Autodesk Fusion 360 part; units mm, degrees
note: some values were not read from the file. Set by a fixed rule: which sketch regions a step uses.
(part 4 of 4)
sketch "Sketch1 (7)" plane through (0, 0, 0) normal (0, 0, 1) x (1, 0, 0) in component "Top/Bottom (1)"
  line L0 (0, 0) -> (160, 0)
  line L1 (160, 0) -> (160, 54)
  line L2 (160, 54) -> (0, 54)
  line L3 (0, 54) -> (0, 0)
  line L4 (0, 51) -> (160, 51) construction
  line L5 (160, 51) -> (160, 48) construction
  line L6 (160, 48) -> (0, 48) construction
  line L7 (0, 48) -> (0, 51) construction
  line L8 (0, 3) -> (160, 3) construction
  line L9 (160, 3) -> (160, 6) construction
  line L10 (160, 6) -> (0, 6) construction
  line L11 (0, 6) -> (0, 3) construction
  line L12 (10, 48) -> (150, 48) construction
  line L13 (150, 48) -> (150, 38) construction
  line L14 (150, 38) -> (10, 38) construction
  line L15 (10, 38) -> (10, 48) construction
  line L16 (0, 38) -> (160, 38) construction
  line L17 (160, 38) -> (160, 36) construction
  line L18 (160, 36) -> (0, 36) construction
  line L19 (0, 36) -> (0, 38) construction
  line L20 (80, 54) -> (80, 0) construction
  point P0 (80, 51)
  point P1 (80, 48)
  point P2 (80, 38)
  point P3 (80, 38)
  point P4 (80, 6)
  dimension "d101_1" = 160
  dimension "d102_1" = 3
  dimension "d103_1" = 3
  dimension "d104_1" = 10
  dimension "d105_1" = 2
  dimension "d106_1" = 140
  dimension "d107_1" = 30
  dimension "d108_1" = 3
  dimension "d109_1" = 3
  constraint horizontal L0
  constraint vertical L1
  constraint horizontal L2
  constraint vertical L3
  constraint coincident L0.start L3.end
  constraint horizontal L4
  constraint vertical L5
  constraint horizontal L6
  constraint vertical L7
  constraint horizontal L8
  constraint vertical L9
  constraint horizontal L10
  constraint vertical L11
  constraint horizontal L12
  constraint vertical L13
  constraint horizontal L14
  constraint vertical L15
  constraint horizontal L16
  constraint vertical L17
  constraint horizontal L18
  constraint vertical L19
  constraint midpoint L2 L20.start
  constraint midpoint L0 L20.end
  constraint midpoint L4 P0
  constraint midpoint L12 P1
  constraint midpoint L16 P3
  constraint midpoint L14 P3
  constraint coincident L20 P0
  constraint coincident P3 P2
  constraint midpoint L10 P4
  constraint coincident L20 P4
  constraint coincident L3 L4.start
  constraint coincident L20 P3
  constraint coincident L6 P1
  constraint coincident L3 L18.end
  constraint coincident L3 L8.start
  measures "d101_1" distance of L17 L19
  measures "d102_1" distance of L2 L4
  measures "d103_1" distance of L4 L6
  measures "d104_1" distance of L12.start L14.end
  measures "d105_1" distance of L16.start L18.end
  measures "d106_1" distance of L13 L15
  measures "d107_1" distance of L10 L18
  measures "d108_1" distance of L8 L10
  measures "d109_1" distance of L0 L8
extrude "Extrude1''''''" add sketch "Sketch1 (7)" along normal blind 10 separate body makes body 7 in component "Top/Bottom (1)"
sketch "Sketch2 (5)" plane through (0, 0, 10) normal (0, 0, 1) x (-1, 0, 0) in component "Top/Bottom (1)"
  line L0 (0, -54) -> (0, 0)
  line L1 (0, 0) -> (-160, 0)
  line L2 (-160, 0) -> (-160, -54)
  line L3 (-160, -54) -> (0, -54)
  line L4 (0, -3) -> (-160, -3)
  line L5 (-160, -6) -> (0, -6)
  line L6 (-160, -48) -> (0, -48)
  line L7 (0, -51) -> (-160, -51)
  line L8 (-79, -48) -> (-81, -48)
  line L9 (-81, -48) -> (-81, -38)
  line L10 (-81, -38) -> (-79, -38)
  line L11 (-79, -38) -> (-79, -48)
  line L12 (-80, -54) -> (-80, 0)
  line L13 (-149, -38) -> (-149, -48)
  line L14 (-151, -48) -> (-151, -38)
  line L15 (-151, -38) -> (-149, -38)
  line L16 (-139, -38) -> (-139, -48)
  line L17 (-141, -48) -> (-141, -38)
  line L18 (-141, -38) -> (-139, -38)
  line L19 (-129, -38) -> (-129, -48)
  line L20 (-131, -48) -> (-131, -38)
  line L21 (-131, -38) -> (-129, -38)
  line L22 (-119, -38) -> (-119, -48)
  line L23 (-121, -48) -> (-121, -38)
  line L24 (-121, -38) -> (-119, -38)
  line L25 (-109, -38) -> (-109, -48)
  line L26 (-111, -48) -> (-111, -38)
  line L27 (-111, -38) -> (-109, -38)
  line L28 (-99, -38) -> (-99, -48)
  line L29 (-101, -48) -> (-101, -38)
  line L30 (-101, -38) -> (-99, -38)
  line L31 (-89, -38) -> (-89, -48)
  line L32 (-91, -48) -> (-91, -38)
  line L33 (-91, -38) -> (-89, -38)
  line L34 (-69, -38) -> (-69, -48)
  line L35 (-71, -48) -> (-71, -38)
  line L36 (-71, -38) -> (-69, -38)
  line L37 (-59, -38) -> (-59, -48)
  line L38 (-61, -48) -> (-61, -38)
  line L39 (-61, -38) -> (-59, -38)
  line L40 (-49, -38) -> (-49, -48)
  line L41 (-51, -48) -> (-51, -38)
  line L42 (-51, -38) -> (-49, -38)
  line L43 (-39, -38) -> (-39, -48)
  line L44 (-41, -48) -> (-41, -38)
  line L45 (-41, -38) -> (-39, -38)
  line L46 (-29, -38) -> (-29, -48)
  line L47 (-31, -48) -> (-31, -38)
  line L48 (-31, -38) -> (-29, -38)
  line L49 (-19, -38) -> (-19, -48)
  line L50 (-21, -48) -> (-21, -38)
  line L51 (-21, -38) -> (-19, -38)
  line L52 (-9, -38) -> (-9, -48)
  line L53 (-11, -48) -> (-11, -38)
  line L54 (-11, -38) -> (-9, -38)
  point P0 (-80, -48)
  dimension "d112_1" = 2
  dimension "d113_1" = 10
  dimension "d116_1" = 10
  dimension "d117_1" = 0
  constraint horizontal L8
  constraint vertical L9
  constraint horizontal L10
  constraint vertical L11
  constraint midpoint L8 P0
  constraint coincident P0 L12
  constraint coincident L6 P0
  measures "d112_1" distance of L8.start L8.end
  measures "d113_1" distance of L8.start L10.end
extrude "Extrude2''''" cut sketch "Sketch2 (5)" against normal blind 5 contours L0 L6 L7 L8 L12 | L2 L6 L7 L8 L12 | L0 L4 L5 L12 | L6 L52 L53 L54 | L6 L8 L10 L11 L12 | L6 L8 L9 L10 L12 | L2 L4 L5 L12 | L6 L49 L50 L51 | L6 L13 L14 L15 | L6 L31 L32 L33 | L6 L34 L35 L36 | L6 L46 L47 L48 | L6 L16 L17 L18 | L6 L28 L29 L30 | L6 L37 L38 L39 | L6 L43 L44 L45 | L6 L19 L20 L21 | L6 L25 L26 L27 | L6 L40 L41 L42 | L6 L22 L23 L24 bodies 7 in component "Top/Bottom (1)"
chamfer "Chamfer1'" distance 1 angle 45 62 edges at (155.5, 48, 10) (151, 43, 10) (150, 38, 10) (145, 48, 10) (141, 43, 10) (140, 38, 10) (139, 43, 10) (131, 43, 10) (130, 38, 10) (129, 43, 10) (135, 48, 10) (125, 48, 10) (121, 43, 10) (120, 38, 10) (119, 43, 10) (115, 48, 10) (111, 43, 10) (110, 38, 10) (109, 43, 10) (105, 48, 10) (101, 43, 10) (99, 43, 10) (100, 38, 10) (91, 43, 10) (95, 48, 10) (89, 43, 10) (90, 38, 10) (81, 43, 10) (79, 43, 10) (80, 38, 10) (75, 48, 10) (85, 48, 10) (69, 43, 10) (71, 43, 10) (70, 38, 10) (61, 43, 10) (59, 43, 10) (60, 38, 10) (51, 43, 10) (49, 43, 10) (50, 38, 10) (55, 48, 10) (65, 48, 10) (45, 48, 10) (41, 43, 10) (40, 38, 10) (39, 43, 10) (35, 48, 10) (29, 43, 10) (31, 43, 10) (30, 38, 10) (21, 43, 10) (20, 38, 10) (19, 43, 10) (11, 43, 10) (10, 38, 10) (9, 43, 10) (15, 48, 10) (4.5, 48, 10) (25, 48, 10) (80, 6, 10) (149, 43, 10) on bodies 7 in component "Top/Bottom (1)"
sketch "Sketch3 (2)" plane through (0, 0, 0) normal (-1, 0, 0) x (0, -1, 0) in component "Top/Bottom (1)"
  line L0 (-6, 9) -> (-7, 10)
  line L1 (-7, 10) -> (-47, 10)
  line L2 (-47, 10) -> (-48, 9)
  line L3 (-48, 9) -> (-48, 5)
  line L4 (-48, 5) -> (-51, 5)
  line L5 (-51, 5) -> (-51, 10)
  line L6 (-51, 10) -> (-54, 10)
  line L7 (-54, 10) -> (-54, 0)
  line L8 (-54, 0) -> (0, 0)
  line L9 (0, 0) -> (0, 10)
  line L10 (0, 10) -> (-3, 10)
  line L11 (-3, 10) -> (-3, 5)
  line L12 (-3, 5) -> (-6, 5)
  line L13 (-6, 5) -> (-6, 9)
  line L14 (-48, 5) -> (-6, 5) construction
  circle A0 centre (-43, 5) radius 1.85
  circle A1 centre (-11, 5) radius 1.85
  circle A2 centre (-43, 5) radius 1.6
  circle A3 centre (-11, 5) radius 1.6
  dimension "d121_1" = 3.7
  dimension "d122_1" = 3.7
  dimension "d123_1" = 5
  dimension "d124_1" = 5
  dimension "d127_1" = 3.2
  dimension "d128_1" = 3.2
  constraint coincident L3.end L4.start
  constraint coincident L12.end L13.start
  constraint coincident L14 A0.centre
  constraint coincident L14 A1.centre
  constraint concentric A0 A2
  constraint concentric A1 A3
  measures "d121_1" diameter of A0
  measures "d122_1" diameter of A1
  measures "d123_1" distance of L3.end A0.centre
  measures "d124_1" distance of L12.end A1.centre
  measures "d127_1" diameter of A2
  measures "d128_1" diameter of A3
sketch "Sketch4 (2)" plane through (160, 0, 0) normal (1, 0, 0) x (0, 1, 0) in component "Top/Bottom (1)"
  line L0 (7, 10) -> (6, 9)
  line L1 (6, 9) -> (6, 5)
  line L2 (6, 5) -> (3, 5)
  line L3 (3, 5) -> (3, 10)
  line L4 (3, 10) -> (0, 10)
  line L5 (0, 10) -> (0, 0)
  line L6 (0, 0) -> (54, 0)
  line L7 (54, 0) -> (54, 10)
  line L8 (54, 10) -> (51, 10)
  line L9 (51, 10) -> (51, 5)
  line L10 (51, 5) -> (48, 5)
  line L11 (48, 5) -> (48, 9)
  line L12 (48, 9) -> (47, 10)
  line L13 (47, 10) -> (7, 10)
  circle A0 centre (11, 5) radius 1.85
  circle A1 centre (11, 5) radius 1.6
  circle A2 centre (43, 5) radius 1.85
  circle A3 centre (43, 5) radius 1.6
extrude "Extrude5'" cut sketch "Sketch4 (2)" against normal blind 15 contours A1 | A3 bodies 7 in component "Top/Bottom (1)"
extrude "Extrude6'" cut sketch "Sketch4 (2)" against normal blind 5 contours A0 | A2 bodies 7 in component "Top/Bottom (1)"
extrude "Extrude7'" cut sketch "Sketch3 (2)" against normal blind 15 contours A2 | A3 bodies 7 in component "Top/Bottom (1)"
extrude "Extrude8'" cut sketch "Sketch3 (2)" against normal blind 5 contours A0 | A1 bodies 7 in component "Top/Bottom (1)"
chamfer "Chamfer2'''" distance 1 angle 45 4 edges at (0, 44.7248, 5.669) (0, 12.7248, 5.669) (160, 41.2752, 5.669) (160, 9.2752, 5.669) on bodies 7 in component "Top/Bottom (1)"
sketch "Sketch1 (8)" plane through (0, 0, 0) normal (0, 0, 1) x (1, 0, 0) in component "Grid"
  line L0 (-5, 9) -> (165, 9)
  line L1 (165, 9) -> (165, 11)
  line L2 (165, 11) -> (-5, 11)
  line L3 (-5, 11) -> (-5, 9)
  line L4 (11, -5) -> (9, -5)
  line L5 (9, -5) -> (9, 165)
  line L6 (9, 165) -> (11, 165)
  line L7 (11, 165) -> (11, -5)
  line L8 (0, 0) -> (228.3171, 0) construction
  line L9 (0, 0) -> (0, 200) construction
  line L10 (19, -5) -> (19, 165)
  line L11 (19, 165) -> (21, 165)
  line L12 (21, 165) -> (21, -5)
  line L13 (21, -5) -> (19, -5)
  line L14 (29, -5) -> (29, 165)
  line L15 (29, 165) -> (31, 165)
  line L16 (31, 165) -> (31, -5)
  line L17 (31, -5) -> (29, -5)
  line L18 (39, -5) -> (39, 165)
  line L19 (39, 165) -> (41, 165)
  line L20 (41, 165) -> (41, -5)
  line L21 (41, -5) -> (39, -5)
  line L22 (49, -5) -> (49, 165)
  line L23 (49, 165) -> (51, 165)
  line L24 (51, 165) -> (51, -5)
  line L25 (51, -5) -> (49, -5)
  line L26 (59, -5) -> (59, 165)
  line L27 (59, 165) -> (61, 165)
  line L28 (61, 165) -> (61, -5)
  line L29 (61, -5) -> (59, -5)
  line L30 (69, -5) -> (69, 165)
  line L31 (69, 165) -> (71, 165)
  line L32 (71, 165) -> (71, -5)
  line L33 (71, -5) -> (69, -5)
  line L34 (79, -5) -> (79, 165)
  line L35 (79, 165) -> (81, 165)
  line L36 (81, 165) -> (81, -5)
  line L37 (81, -5) -> (79, -5)
  line L38 (89, -5) -> (89, 165)
  line L39 (89, 165) -> (91, 165)
  line L40 (91, 165) -> (91, -5)
  line L41 (91, -5) -> (89, -5)
  line L42 (99, -5) -> (99, 165)
  line L43 (99, 165) -> (101, 165)
  line L44 (101, 165) -> (101, -5)
  line L45 (101, -5) -> (99, -5)
  line L46 (109, -5) -> (109, 165)
  line L47 (109, 165) -> (111, 165)
  line L48 (111, 165) -> (111, -5)
  line L49 (111, -5) -> (109, -5)
  line L50 (119, -5) -> (119, 165)
  line L51 (119, 165) -> (121, 165)
  line L52 (121, 165) -> (121, -5)
  line L53 (121, -5) -> (119, -5)
  line L54 (129, -5) -> (129, 165)
  line L55 (129, 165) -> (131, 165)
  line L56 (131, 165) -> (131, -5)
  line L57 (131, -5) -> (129, -5)
  line L58 (139, -5) -> (139, 165)
  line L59 (139, 165) -> (141, 165)
  line L60 (141, 165) -> (141, -5)
  line L61 (141, -5) -> (139, -5)
  line L62 (149, -5) -> (149, 165)
  line L63 (149, 165) -> (151, 165)
  line L64 (151, 165) -> (151, -5)
  line L65 (151, -5) -> (149, -5)
  line L66 (165, 21) -> (-5, 21)
  line L67 (-5, 21) -> (-5, 19)
  line L68 (-5, 19) -> (165, 19)
  line L69 (165, 19) -> (165, 21)
  line L70 (165, 31) -> (-5, 31)
  line L71 (-5, 31) -> (-5, 29)
  line L72 (-5, 29) -> (165, 29)
  line L73 (165, 29) -> (165, 31)
  line L74 (165, 41) -> (-5, 41)
  line L75 (-5, 41) -> (-5, 39)
  line L76 (-5, 39) -> (165, 39)
  line L77 (165, 39) -> (165, 41)
  line L78 (165, 51) -> (-5, 51)
  line L79 (-5, 51) -> (-5, 49)
  line L80 (-5, 49) -> (165, 49)
  line L81 (165, 49) -> (165, 51)
  line L82 (165, 61) -> (-5, 61)
  line L83 (-5, 61) -> (-5, 59)
  line L84 (-5, 59) -> (165, 59)
  line L85 (165, 59) -> (165, 61)
  line L86 (165, 71) -> (-5, 71)
  line L87 (-5, 71) -> (-5, 69)
  line L88 (-5, 69) -> (165, 69)
  line L89 (165, 69) -> (165, 71)
  line L90 (165, 81) -> (-5, 81)
  line L91 (-5, 81) -> (-5, 79)
  line L92 (-5, 79) -> (165, 79)
  line L93 (165, 79) -> (165, 81)
  line L94 (165, 91) -> (-5, 91)
  line L95 (-5, 91) -> (-5, 89)
  line L96 (-5, 89) -> (165, 89)
  line L97 (165, 89) -> (165, 91)
  line L98 (165, 101) -> (-5, 101)
  line L99 (-5, 101) -> (-5, 99)
  line L100 (-5, 99) -> (165, 99)
  line L101 (165, 99) -> (165, 101)
  line L102 (165, 111) -> (-5, 111)
  line L103 (-5, 111) -> (-5, 109)
  line L104 (-5, 109) -> (165, 109)
  line L105 (165, 109) -> (165, 111)
  line L106 (165, 121) -> (-5, 121)
  line L107 (-5, 121) -> (-5, 119)
  line L108 (-5, 119) -> (165, 119)
  line L109 (165, 119) -> (165, 121)
  line L110 (165, 131) -> (-5, 131)
  line L111 (-5, 131) -> (-5, 129)
  line L112 (-5, 129) -> (165, 129)
  line L113 (165, 129) -> (165, 131)
  line L114 (165, 141) -> (-5, 141)
  line L115 (-5, 141) -> (-5, 139)
  line L116 (-5, 139) -> (165, 139)
  line L117 (165, 139) -> (165, 141)
  line L118 (165, 151) -> (-5, 151)
  line L119 (-5, 151) -> (-5, 149)
  line L120 (-5, 149) -> (165, 149)
  line L121 (165, 149) -> (165, 151)
  point P0 (0, 9)
  point P1 (9, 0)
  point P2 (10, -5)
  point P3 (-5, 10)
  dimension "d140" = 170
  dimension "d141" = 2
  dimension "d142" = 170
  dimension "d143" = 2
  dimension "d144" = 5
  dimension "d145" = 5
  dimension "d146" = 9
  dimension "d147" = 9
  dimension "d150" = 10
  dimension "d151" = 0
  dimension "d154" = 0
  dimension "d155" = 10
  constraint horizontal L0
  constraint vertical L1
  constraint horizontal L2
  constraint vertical L3
  constraint horizontal L4
  constraint vertical L5
  constraint horizontal L6
  constraint vertical L7
  constraint coincident L8.start L9.start
  constraint perpendicular L5 L8
  constraint perpendicular L8 L9
  constraint coincident L0 P0
  constraint coincident L5 P1
  constraint midpoint L4 P2
  constraint midpoint L3 P3
  constraint coincident L9 P0
  constraint coincident L8 P1
  measures "d140" distance of L0.start L0.end
  measures "d141" distance of L0.start L2.end
  measures "d142" distance of L4.end L5.end
  measures "d143" distance of L5.end L6.end
  measures "d144" distance of L3 P0
  measures "d145" distance of L4 P1
  measures "d146" distance of L8.start P1
  measures "d147" distance of L8.start L0
extrude "Extrude1'''''''" add sketch "Sketch1 (8)" along normal blind 10 separate body contours L0 L2 L3 L5 | L0 L2 L5 L7 | L0 L4 L5 L7 | L0 L2 L7 L10 | L2 L5 L7 L68 | L0 L2 L10 L12 | L0 L10 L12 L13 | L5 L66 L67 L68 | L5 L7 L66 L68 | L0 L2 L12 L14 | L2 L10 L12 L68 | L7 L10 L66 L68 | L5 L7 L66 L72 | L0 L2 L14 L16 | L0 L14 L16 L17 | L10 L12 L66 L68 | L5 L70 L71 L72 | L5 L7 L70 L72 | L0 L2 L16 L18 | L2 L14 L16 L68 | L12 L14 L66 L68 | L10 L12 L66 L72 | L7 L10 L70 L72 | L5 L7 L70 L76 | L0 L2 L18 L20 | L0 L18 L20 L21 | L14 L16 L66 L68 | L10 L12 L70 L72 | L5 L74 L75 L76 | L5 L7 L74 L76 | L0 L2 L20 L22 | L2 L18 L20 L68 | L16 L18 L66 L68 | L14 L16 L66 L72 | L12 L14 L70 L72 | L10 L12 L70 L76 | L7 L10 L74 L76 | L5 L7 L74 L80 | L0 L2 L22 L24 | L0 L22 L24 L25 | L18 L20 L66 L68 | L14 L16 L70 L72 | L10 L12 L74 L76 | L5 L78 L79 L80 | L5 L7 L78 L80 | L0 L2 L24 L26 | L2 L22 L24 L68 | L20 L22 L66 L68 | L18 L20 L66 L72 | L16 L18 L70 L72 | L14 L16 L70 L76 | L12 L14 L74 L76 | L10 L12 L74 L80 | L7 L10 L78 L80 | L5 L7 L78 L84 | L0 L2 L26 L28 | L0 L26 L28 L29 | L22 L24 L66 L68 | L18 L20 L70 L72 | L14 L16 L74 L76 | L10 L12 L78 L80 | L5 L82 L83 L84 | L5 L7 L82 L84 | L0 L2 L28 L30 | L2 L26 L28 L68 | L24 L26 L66 L68 | L22 L24 L66 L72 | L20 L22 L70 L72 | L18 L20 L70 L76 | L16 L18 L74 L76 | L14 L16 L74 L80 | L12 L14 L78 L80 | L10 L12 L78 L84 | L7 L10 L82 L84 | L5 L7 L82 L88 | L0 L2 L30 L32 | L0 L30 L32 L33 | L26 L28 L66 L68 | L22 L24 L70 L72 | L18 L20 L74 L76 | L14 L16 L78 L80 | L10 L12 L82 L84 | L5 L86 L87 L88 | L5 L7 L86 L88 | L0 L2 L32 L34 | L2 L30 L32 L68 | L28 L30 L66 L68 | L26 L28 L66 L72 | L24 L26 L70 L72 | L22 L24 L70 L76 | L20 L22 L74 L76 | L18 L20 L74 L80 | L16 L18 L78 L80 | L14 L16 L78 L84 | L12 L14 L82 L84 | L10 L12 L82 L88 | L7 L10 L86 L88 | L5 L7 L86 L92 | L0 L2 L34 L36 | L0 L34 L36 L37 | L30 L32 L66 L68 | L26 L28 L70 L72 | L22 L24 L74 L76 | L18 L20 L78 L80 | L14 L16 L82 L84 | L10 L12 L86 L88 | L5 L90 L91 L92 | L5 L7 L90 L92 | L0 L2 L36 L38 | L2 L34 L36 L68 | L32 L34 L66 L68 | L30 L32 L66 L72 | L28 L30 L70 L72 | L26 L28 L70 L76 | L24 L26 L74 L76 | L22 L24 L74 L80 | L20 L22 L78 L80 | L18 L20 L78 L84 | L16 L18 L82 L84 | L14 L16 L82 L88 | L12 L14 L86 L88 | L10 L12 L86 L92 | L7 L10 L90 L92 | L5 L7 L90 L96 | L0 L2 L38 L40 | L0 L38 L40 L41 | L34 L36 L66 L68 | L30 L32 L70 L72 | L26 L28 L74 L76 | L22 L24 L78 L80 | L18 L20 L82 L84 | L14 L16 L86 L88 | L10 L12 L90 L92 | L5 L94 L95 L96 | L5 L7 L94 L96 | L0 L2 L40 L42 | L2 L38 L40 L68 | L36 L38 L66 L68 | L34 L36 L66 L72 | L32 L34 L70 L72 | L30 L32 L70 L76 | L28 L30 L74 L76 | L26 L28 L74 L80 | L24 L26 L78 L80 | L22 L24 L78 L84 | L20 L22 L82 L84 | L18 L20 L82 L88 | L16 L18 L86 L88 | L14 L16 L86 L92 | L12 L14 L90 L92 | L10 L12 L90 L96 | L7 L10 L94 L96 | L5 L7 L94 L100 | L0 L2 L42 L44 | L0 L42 L44 L45 | L38 L40 L66 L68 | L34 L36 L70 L72 | L30 L32 L74 L76 | L26 L28 L78 L80 | L22 L24 L82 L84 | L18 L20 L86 L88 | L14 L16 L90 L92 | L10 L12 L94 L96 | L5 L98 L99 L100 | L5 L7 L98 L100 | L0 L2 L44 L46 | L2 L42 L44 L68 | L40 L42 L66 L68 | L38 L40 L66 L72 | L36 L38 L70 L72 | L34 L36 L70 L76 | L32 L34 L74 L76 | L30 L32 L74 L80 | L28 L30 L78 L80 | L26 L28 L78 L84 | L24 L26 L82 L84 | L22 L24 L82 L88 | L20 L22 L86 L88 | L18 L20 L86 L92 | L16 L18 L90 L92 | L14 L16 L90 L96 | L12 L14 L94 L96 | L10 L12 L94 L100 | L7 L10 L98 L100 | L5 L7 L98 L104 | L0 L2 L46 L48 | L0 L46 L48 L49 | L42 L44 L66 L68 | L38 L40 L70 L72 | L34 L36 L74 L76 | L30 L32 L78 L80 | L26 L28 L82 L84 | L22 L24 L86 L88 | L18 L20 L90 L92 | L14 L16 L94 L96 | L10 L12 L98 L100 | L5 L102 L103 L104 | L5 L7 L102 L104 | L0 L2 L48 L50 | L2 L46 L48 L68 | L44 L46 L66 L68 | L42 L44 L66 L72 | L40 L42 L70 L72 | L38 L40 L70 L76 | L36 L38 L74 L76 | L34 L36 L74 L80 | L32 L34 L78 L80 | L30 L32 L78 L84 | L28 L30 L82 L84 | L26 L28 L82 L88 | L24 L26 L86 L88 | L22 L24 L86 L92 | L20 L22 L90 L92 | L18 L20 L90 L96 | L16 L18 L94 L96 | L14 L16 L94 L100 | L12 L14 L98 L100 | L10 L12 L98 L104 | L7 L10 L102 L104 | L5 L7 L102 L108 | L0 L2 L50 L52 | L0 L50 L52 L53 | L46 L48 L66 L68 | L42 L44 L70 L72 | L38 L40 L74 L76 | L34 L36 L78 L80 | L30 L32 L82 L84 | L26 L28 L86 L88 | L22 L24 L90 L92 | L18 L20 L94 L96 | L14 L16 L98 L100 | L10 L12 L102 L104 | L5 L106 L107 L108 | L5 L7 L106 L108 | L0 L2 L52 L54 | L2 L50 L52 L68 | L48 L50 L66 L68 | L46 L48 L66 L72 | L44 L46 L70 L72 | L42 L44 L70 L76 | L40 L42 L74 L76 | L38 L40 L74 L80 | L36 L38 L78 L80 | L34 L36 L78 L84 | L32 L34 L82 L84 | L30 L32 L82 L88 | L28 L30 L86 L88 | L26 L28 L86 L92 | L24 L26 L90 L92 | L22 L24 L90 L96 | L20 L22 L94 L96 | L18 L20 L94 L100 | L16 L18 L98 L100 | L14 L16 L98 L104 | L12 L14 L102 L104 | L10 L12 L102 L108 | L7 L10 L106 L108 | L5 L7 L106 L112 | L0 L2 L54 L56 | L0 L54 L56 L57 | L50 L52 L66 L68 | L46 L48 L70 L72 | L42 L44 L74 L76 | L38 L40 L78 L80 | L34 L36 L82 L84 | L30 L32 L86 L88 | L26 L28 L90 L92 | L22 L24 L94 L96 | L18 L20 L98 L100 | L14 L16 L102 L104 | L10 L12 L106 L108 | L5 L110 L111 L112 | L5 L7 L110 L112 | L0 L2 L56 L58 | L2 L54 L56 L68 | L52 L54 L66 L68 | L50 L52 L66 L72 | L48 L50 L70 L72 | L46 L48 L70 L76 | L44 L46 L74 L76 | L42 L44 L74 L80 | L40 L42 L78 L80 | L38 L40 L78 L84 | L36 L38 L82 L84 | L34 L36 L82 L88 | L32 L34 L86 L88 | L30 L32 L86 L92 | L28 L30 L90 L92 | L26 L28 L90 L96 | L24 L26 L94 L96 | L22 L24 L94 L100 | L20 L22 L98 L100 | L18 L20 L98 L104 | L16 L18 L102 L104 | L14 L16 L102 L108 | L12 L14 L106 L108 | L10 L12 L106 L112 | L7 L10 L110 L112 | L5 L7 L110 L116 | L0 L2 L58 L60 | L0 L58 L60 L61 | L54 L56 L66 L68 | L50 L52 L70 L72 | L46 L48 L74 L76 | L42 L44 L78 L80 | L38 L40 L82 L84 | L34 L36 L86 L88 | L30 L32 L90 L92 | L26 L28 L94 L96 | L22 L24 L98 L100 | L18 L20 L102 L104 | L14 L16 L106 L108 | L10 L12 L110 L112 | L5 L114 L115 L116 | L5 L7 L114 L116 | L0 L2 L60 L62 | L2 L58 L60 L68 | L56 L58 L66 L68 | L54 L56 L66 L72 | L52 L54 L70 L72 | L50 L52 L70 L76 | L48 L50 L74 L76 | L46 L48 L74 L80 | L44 L46 L78 L80 | L42 L44 L78 L84 | L40 L42 L82 L84 | L38 L40 L82 L88 | L36 L38 L86 L88 | L34 L36 L86 L92 | L32 L34 L90 L92 | L30 L32 L90 L96 | L28 L30 L94 L96 | L26 L28 L94 L100 | L24 L26 L98 L100 | L22 L24 L98 L104 | L20 L22 L102 L104 | L18 L20 L102 L108 | L16 L18 L106 L108 | L14 L16 L106 L112 | L12 L14 L110 L112 | L10 L12 L110 L116 | L7 L10 L114 L116 | L5 L7 L114 L120 | L0 L2 L62 L64 | L0 L62 L64 L65 | L58 L60 L66 L68 | L54 L56 L70 L72 | L50 L52 L74 L76 | L46 L48 L78 L80 | L42 L44 L82 L84 | L38 L40 L86 L88 | L34 L36 L90 L92 | L30 L32 L94 L96 | L26 L28 L98 L100 | L22 L24 L102 L104 | L18 L20 L106 L108 | L14 L16 L110 L112 | L10 L12 L114 L116 | L5 L118 L119 L120 | L5 L7 L118 L120 | L0 L1 L2 L64 | L2 L62 L64 L68 | L60 L62 L66 L68 | L58 L60 L66 L72 | L56 L58 L70 L72 | L54 L56 L70 L76 | L52 L54 L74 L76 | L50 L52 L74 L80 | L48 L50 L78 L80 | L46 L48 L78 L84 | L44 L46 L82 L84 | L42 L44 L82 L88 | L40 L42 L86 L88 | L38 L40 L86 L92 | L36 L38 L90 L92 | L34 L36 L90 L96 | L32 L34 L94 L96 | L30 L32 L94 L100 | L28 L30 L98 L100 | L26 L28 L98 L104 | L24 L26 L102 L104 | L22 L24 L102 L108 | L20 L22 L106 L108 | L18 L20 L106 L112 | L16 L18 L110 L112 | L14 L16 L110 L116 | L12 L14 L114 L116 | L10 L12 L114 L120 | L7 L10 L118 L120 | L5 L6 L7 L118 | L62 L64 L66 L68 | L58 L60 L70 L72 | L54 L56 L74 L76 | L50 L52 L78 L80 | L46 L48 L82 L84 | L42 L44 L86 L88 | L38 L40 L90 L92 | L34 L36 L94 L96 | L30 L32 L98 L100 | L26 L28 L102 L104 | L22 L24 L106 L108 | L18 L20 L110 L112 | L14 L16 L114 L116 | L10 L12 L118 L120 | L64 L66 L68 L69 | L62 L64 L66 L72 | L60 L62 L70 L72 | L58 L60 L70 L76 | L56 L58 L74 L76 | L54 L56 L74 L80 | L52 L54 L78 L80 | L50 L52 L78 L84 | L48 L50 L82 L84 | L46 L48 L82 L88 | L44 L46 L86 L88 | L42 L44 L86 L92 | L40 L42 L90 L92 | L38 L40 L90 L96 | L36 L38 L94 L96 | L34 L36 L94 L100 | L32 L34 L98 L100 | L30 L32 L98 L104 | L28 L30 L102 L104 | L26 L28 L102 L108 | L24 L26 L106 L108 | L22 L24 L106 L112 | L20 L22 L110 L112 | L18 L20 L110 L116 | L16 L18 L114 L116 | L14 L16 L114 L120 | L12 L14 L118 L120 | L10 L11 L12 L118 | L62 L64 L70 L72 | L58 L60 L74 L76 | L54 L56 L78 L80 | L50 L52 L82 L84 | L46 L48 L86 L88 | L42 L44 L90 L92 | L38 L40 L94 L96 | L34 L36 L98 L100 | L30 L32 L102 L104 | L26 L28 L106 L108 | L22 L24 L110 L112 | L18 L20 L114 L116 | L14 L16 L118 L120 | L64 L70 L72 L73 | L62 L64 L70 L76 | L60 L62 L74 L76 | L58 L60 L74 L80 | L56 L58 L78 L80 | L54 L56 L78 L84 | L52 L54 L82 L84 | L50 L52 L82 L88 | L48 L50 L86 L88 | L46 L48 L86 L92 | L44 L46 L90 L92 | L42 L44 L90 L96 | L40 L42 L94 L96 | L38 L40 L94 L100 | L36 L38 L98 L100 | L34 L36 L98 L104 | L32 L34 L102 L104 | L30 L32 L102 L108 | L28 L30 L106 L108 | L26 L28 L106 L112 | L24 L26 L110 L112 | L22 L24 L110 L116 | L20 L22 L114 L116 | L18 L20 L114 L120 | L16 L18 L118 L120 | L14 L15 L16 L118 | L62 L64 L74 L76 | L58 L60 L78 L80 | L54 L56 L82 L84 | L50 L52 L86 L88 | L46 L48 L90 L92 | L42 L44 L94 L96 | L38 L40 L98 L100 | L34 L36 L102 L104 | L30 L32 L106 L108 | L26 L28 L110 L112 | L22 L24 L114 L116 | L18 L20 L118 L120 | L64 L74 L76 L77 | L62 L64 L74 L80 | L60 L62 L78 L80 | L58 L60 L78 L84 | L56 L58 L82 L84 | L54 L56 L82 L88 | L52 L54 L86 L88 | L50 L52 L86 L92 | L48 L50 L90 L92 | L46 L48 L90 L96 | L44 L46 L94 L96 | L42 L44 L94 L100 | L40 L42 L98 L100 | L38 L40 L98 L104 | L36 L38 L102 L104 | L34 L36 L102 L108 | L32 L34 L106 L108 | L30 L32 L106 L112 | L28 L30 L110 L112 | L26 L28 L110 L116 | L24 L26 L114 L116 | L22 L24 L114 L120 | L20 L22 L118 L120 | L18 L19 L20 L118 | L62 L64 L78 L80 | L58 L60 L82 L84 | L54 L56 L86 L88 | L50 L52 L90 L92 | L46 L48 L94 L96 | L42 L44 L98 L100 | L38 L40 L102 L104 | L34 L36 L106 L108 | L30 L32 L110 L112 | L26 L28 L114 L116 | L22 L24 L118 L120 | L64 L78 L80 L81 | L62 L64 L78 L84 | L60 L62 L82 L84 | L58 L60 L82 L88 | L56 L58 L86 L88 | L54 L56 L86 L92 | L52 L54 L90 L92 | L50 L52 L90 L96 | L48 L50 L94 L96 | L46 L48 L94 L100 | L44 L46 L98 L100 | L42 L44 L98 L104 | L40 L42 L102 L104 | L38 L40 L102 L108 | L36 L38 L106 L108 | L34 L36 L106 L112 | L32 L34 L110 L112 | L30 L32 L110 L116 | L28 L30 L114 L116 | L26 L28 L114 L120 | L24 L26 L118 L120 | L22 L23 L24 L118 | L62 L64 L82 L84 | L58 L60 L86 L88 | L54 L56 L90 L92 | L50 L52 L94 L96 | L46 L48 L98 L100 | L42 L44 L102 L104 | L38 L40 L106 L108 | L34 L36 L110 L112 | L30 L32 L114 L116 | L26 L28 L118 L120 | L64 L82 L84 L85 | L62 L64 L82 L88 | L60 L62 L86 L88 | L58 L60 L86 L92 | L56 L58 L90 L92 | L54 L56 L90 L96 | L52 L54 L94 L96 | L50 L52 L94 L100 | L48 L50 L98 L100 | L46 L48 L98 L104 | L44 L46 L102 L104 | L42 L44 L102 L108 | L40 L42 L106 L108 | L38 L40 L106 L112 | L36 L38 L110 L112 | L34 L36 L110 L116 | L32 L34 L114 L116 | L30 L32 L114 L120 | L28 L30 L118 L120 | L26 L27 L28 L118 | L62 L64 L86 L88 | L58 L60 L90 L92 | L54 L56 L94 L96 | L50 L52 L98 L100 | L46 L48 L102 L104 | L42 L44 L106 L108 | L38 L40 L110 L112 | L34 L36 L114 L116 | L30 L32 L118 L120 | L64 L86 L88 L89 | L62 L64 L86 L92 | L60 L62 L90 L92 | L58 L60 L90 L96 | L56 L58 L94 L96 | L54 L56 L94 L100 | L52 L54 L98 L100 | L50 L52 L98 L104 | L48 L50 L102 L104 | L46 L48 L102 L108 | L44 L46 L106 L108 | L42 L44 L106 L112 | L40 L42 L110 L112 | L38 L40 L110 L116 | L36 L38 L114 L116 | L34 L36 L114 L120 | L32 L34 L118 L120 | L30 L31 L32 L118 | L62 L64 L90 L92 | L58 L60 L94 L96 | L54 L56 L98 L100 | L50 L52 L102 L104 | L46 L48 L106 L108 | L42 L44 L110 L112 | L38 L40 L114 L116 | L34 L36 L118 L120 | L64 L90 L92 L93 | L62 L64 L90 L96 | L60 L62 L94 L96 | L58 L60 L94 L100 | L56 L58 L98 L100 | L54 L56 L98 L104 | L52 L54 L102 L104 | L50 L52 L102 L108 | L48 L50 L106 L108 | L46 L48 L106 L112 | L44 L46 L110 L112 | L42 L44 L110 L116 | L40 L42 L114 L116 | L38 L40 L114 L120 | L36 L38 L118 L120 | L34 L35 L36 L118 | L62 L64 L94 L96 | L58 L60 L98 L100 | L54 L56 L102 L104 | L50 L52 L106 L108 | L46 L48 L110 L112 | L42 L44 L114 L116 | L38 L40 L118 L120 | L64 L94 L96 L97 | L62 L64 L94 L100 | L60 L62 L98 L100 | L58 L60 L98 L104 | L56 L58 L102 L104 | L54 L56 L102 L108 | L52 L54 L106 L108 | L50 L52 L106 L112 | L48 L50 L110 L112 | L46 L48 L110 L116 | L44 L46 L114 L116 | L42 L44 L114 L120 | L40 L42 L118 L120 | L38 L39 L40 L118 | L62 L64 L98 L100 | L58 L60 L102 L104 | L54 L56 L106 L108 | L50 L52 L110 L112 | L46 L48 L114 L116 | L42 L44 L118 L120 | L64 L98 L100 L101 | L62 L64 L98 L104 | L60 L62 L102 L104 | L58 L60 L102 L108 | L56 L58 L106 L108 | L54 L56 L106 L112 | L52 L54 L110 L112 | L50 L52 L110 L116 | L48 L50 L114 L116 | L46 L48 L114 L120 | L44 L46 L118 L120 | L42 L43 L44 L118 | L62 L64 L102 L104 | L58 L60 L106 L108 | L54 L56 L110 L112 | L50 L52 L114 L116 | L46 L48 L118 L120 | L64 L102 L104 L105 | L62 L64 L102 L108 | L60 L62 L106 L108 | L58 L60 L106 L112 | L56 L58 L110 L112 | L54 L56 L110 L116 | L52 L54 L114 L116 | L50 L52 L114 L120 | L48 L50 L118 L120 | L46 L47 L48 L118 | L62 L64 L106 L108 | L58 L60 L110 L112 | L54 L56 L114 L116 | L50 L52 L118 L120 | L64 L106 L108 L109 | L62 L64 L106 L112 | L60 L62 L110 L112 | L58 L60 L110 L116 | L56 L58 L114 L116 | L54 L56 L114 L120 | L52 L54 L118 L120 | L50 L51 L52 L118 | L62 L64 L110 L112 | L58 L60 L114 L116 | L54 L56 L118 L120 | L64 L110 L112 L113 | L62 L64 L110 L116 | L60 L62 L114 L116 | L58 L60 L114 L120 | L56 L58 L118 L120 | L54 L55 L56 L118 | L62 L64 L114 L116 | L58 L60 L118 L120 | L64 L114 L116 L117 | L62 L64 L114 L120 | L60 L62 L118 L120 | L58 L59 L60 L118 | L62 L64 L118 L120 | L64 L118 L120 L121 | L62 L63 L64 L118 makes body 8 in component "Grid"
move_body "Move1" bodies 7 to x (0, 1, 0) y (0, 0, 1) z (1, 0, 0) at (-5, -5, 0) in component "Top/Bottom (1)"
move_body "Move1'" bodies 6 to x (0, -1, 0) y (0, 0, 1) z (-1, 0, 0) at (-160, 202.4, 0) in component "Top/Bottom"
move_body "Move2" bodies 6 to x (1, 0, 0) y (0, 1, 0) z (0, 0, 1) at (-5, 82.6, 0) in component "Top/Bottom"
move_body "Move3" bodies 6 to x (1, 0, 0) y (0, 1, 0) z (0, 0, 1) at (0, 0, 0) in component "Top/Bottom"
move_body "Move2'" bodies 7 to x (0, -1, 0) y (1, 0, 0) z (0, 0, 1) at (0, 130, 0) in component "Top/Bottom (1)"
move_body "Move4" bodies 6 to x (0, -1, 0) y (1, 0, 0) z (0, 0, 1) at (-180, 100, 0) in component "Top/Bottom"
sketch "Sketch2 (6)" plane through (9, 0, 0) normal (-1, 0, 0) x (0, -1, 0) in component "Grid"
  line L0 (-165, 0) -> (-151, 0)
  line L1 (-151, 0) -> (-151, 10)
  line L2 (-151, 10) -> (-165, 10)
  line L3 (-165, 10) -> (-165, 0)
  line L4 (-1.75, 0) -> (-5.75, 0)
  line L5 (-5.75, 0) -> (-5.75, 2)
  line L6 (-5.75, 2) -> (-1.75, 2)
  line L7 (-1.75, 2) -> (-1.75, 0)
  line L8 (-5, 0) -> (-2.5, 0)
  line L9 (-2.5, 0) -> (-2.5, 1) construction
  line L10 (-2.5, 1) -> (-5, 1) construction
  line L11 (-5, 1) -> (-5, 0) construction
  line L12 (-9, 0) -> (-9, 10) construction
  line L13 (-11, 0) -> (-9, 0) construction
  line L14 (-9, 0) -> (-9, 10)
  line L15 (-9, 10) -> (-11, 10) construction
  line L16 (-11, 10) -> (-11, 0) construction
  line L17 (-15.75, 2) -> (-11.75, 2)
  line L18 (-15.75, 0) -> (-15.75, 2)
  line L19 (-11.75, 2) -> (-11.75, 0)
  line L20 (-11.75, 0) -> (-15.75, 0)
  line L21 (-25.75, 2) -> (-21.75, 2)
  line L22 (-25.75, 0) -> (-25.75, 2)
  line L23 (-21.75, 2) -> (-21.75, 0)
  line L24 (-21.75, 0) -> (-25.75, 0)
  line L25 (-35.75, 2) -> (-31.75, 2)
  line L26 (-35.75, 0) -> (-35.75, 2)
  line L27 (-31.75, 2) -> (-31.75, 0)
  line L28 (-31.75, 0) -> (-35.75, 0)
  line L29 (-45.75, 2) -> (-41.75, 2)
  line L30 (-45.75, 0) -> (-45.75, 2)
  line L31 (-41.75, 2) -> (-41.75, 0)
  line L32 (-41.75, 0) -> (-45.75, 0)
  line L33 (-55.75, 2) -> (-51.75, 2)
  line L34 (-55.75, 0) -> (-55.75, 2)
  line L35 (-51.75, 2) -> (-51.75, 0)
  line L36 (-51.75, 0) -> (-55.75, 0)
  line L37 (-65.75, 2) -> (-61.75, 2)
  line L38 (-65.75, 0) -> (-65.75, 2)
  line L39 (-61.75, 2) -> (-61.75, 0)
  line L40 (-61.75, 0) -> (-65.75, 0)
  line L41 (-75.75, 2) -> (-71.75, 2)
  line L42 (-75.75, 0) -> (-75.75, 2)
  line L43 (-71.75, 2) -> (-71.75, 0)
  line L44 (-71.75, 0) -> (-75.75, 0)
  line L45 (-85.75, 2) -> (-81.75, 2)
  line L46 (-85.75, 0) -> (-85.75, 2)
  line L47 (-81.75, 2) -> (-81.75, 0)
  line L48 (-81.75, 0) -> (-85.75, 0)
  line L49 (-95.75, 2) -> (-91.75, 2)
  line L50 (-95.75, 0) -> (-95.75, 2)
  line L51 (-91.75, 2) -> (-91.75, 0)
  line L52 (-91.75, 0) -> (-95.75, 0)
  line L53 (-105.75, 2) -> (-101.75, 2)
  line L54 (-105.75, 0) -> (-105.75, 2)
  line L55 (-101.75, 2) -> (-101.75, 0)
  line L56 (-101.75, 0) -> (-105.75, 0)
  line L57 (-115.75, 2) -> (-111.75, 2)
  line L58 (-115.75, 0) -> (-115.75, 2)
  line L59 (-111.75, 2) -> (-111.75, 0)
  line L60 (-111.75, 0) -> (-115.75, 0)
  line L61 (-125.75, 2) -> (-121.75, 2)
  line L62 (-125.75, 0) -> (-125.75, 2)
  line L63 (-121.75, 2) -> (-121.75, 0)
  line L64 (-121.75, 0) -> (-125.75, 0)
  line L65 (-135.75, 2) -> (-131.75, 2)
  line L66 (-135.75, 0) -> (-135.75, 2)
  line L67 (-131.75, 2) -> (-131.75, 0)
  line L68 (-131.75, 0) -> (-135.75, 0)
  line L69 (-145.75, 2) -> (-141.75, 2)
  line L70 (-145.75, 0) -> (-145.75, 2)
  line L71 (-141.75, 2) -> (-141.75, 0)
  line L72 (-141.75, 0) -> (-145.75, 0)
  line L73 (-155.75, 2) -> (-151.75, 2)
  line L74 (-155.75, 0) -> (-155.75, 2)
  line L75 (-151.75, 2) -> (-151.75, 0)
  line L76 (-151.75, 0) -> (-155.75, 0)
  point P0 (-3.75, 0)
  point P1 (-3.75, 1)
  dimension "d158" = 2
  dimension "d159" = 4
  dimension "d160" = 5.25
  dimension "d163" = -10
  dimension "d164" = 0
  constraint horizontal L4
  constraint vertical L5
  constraint horizontal L6
  constraint vertical L7
  constraint midpoint L4 P0
  constraint midpoint L10 P1
  constraint horizontal P0 L12.start
  measures "d158" distance of L4.start L6.end
  measures "d159" distance of L5.end L6.end
  measures "d160" distance of P0 L12
extrude "Extrude2'''''" cut sketch "Sketch2 (6)" against normal blind 142 contours L0 L73 L74 L75 L76 | L4 L5 L6 L7 L8 | L17 L18 L19 L20 | L21 L22 L23 L24 | L25 L26 L27 L28 | L29 L30 L31 L32 | L33 L34 L35 L36 | L37 L38 L39 L40 | L41 L42 L43 L44 | L45 L46 L47 L48 | L49 L50 L51 L52 | L53 L54 L55 L56 | L57 L58 L59 L60 | L61 L62 L63 L64 | L65 L66 L67 L68 | L69 L70 L71 L72 bodies 8 in component "Grid"
component "LED_Pannel" placed x (1, 0, 0) y (0, 1, 0) z (0, 0, 1) at (10, 10, 37.8)
component "Diffusion" placed x (1, 0, 0) y (0, 1, 0) z (0, 0, 1) at (5, 5, 48)
component "Backing" placed x (1, 0, 0) y (0, 1, 0) z (0, 0, 1) at (5, 5, 3)
component "Side(holes)" placed x (0, 1, 0) y (0, 0, 1) z (1, 0, 0) at (0, 0, 0)
component "Side(no holes)" placed x (0, -1, 0) y (0, 0, 1) z (-1, 0, 0) at (180, 180, 0)
component "Top/Bottom" placed x (1, 0, 0) y (0, 1, 0) z (0, 0, 1) at (65, -265, 0)
component "Top/Bottom (1)" placed x (1, 0, 0) y (0, 1, 0) z (0, 0, 1) at (15, 45, 0)
component "Grid" placed x (1, 0, 0) y (0, 1, 0) z (0, 0, 1) at (10, 10, 38)
equation "d31 = d77 / 2"
equation "d32 = d31"
equation "d35 = 3 mm + 3 mm + 4 mm"
equation "d36 = d34"
equation "d37 = d34"
equation "d38 = d34"
equation "d42 = 5 mm + 5 mm"
equation "d44 = 160 mm + 10 mm"
equation "d47 = d44"
equation "d48 = d45"
equation "d49 = d46"
equation "d57 = 3 mm + 3 mm"
equation "d70 = d69"
equation "d71 = d68"
equation "d73 = d72"
equation "d74 = 10 mm + 2 mm"
equation "d78 = d77 / 2"
equation "d79 = d78"
equation "d80 = d78"
equation "d81 = d78"
equation "d88 = d87"
equation "d89 = d87"
equation "d98 = -10.00 mm + 2 mm"
equation "d31_1 = d77_1 / 2"
equation "d32_1 = d31_1"
equation "d36_1 = d34_1"
equation "d37_1 = d34_1"
equation "d38_1 = d34_1"
equation "d42_1 = 5 mm + 5 mm"
equation "d47_1 = d44_1"
equation "d48_1 = d45_1"
equation "d49_1 = d46_1"
equation "d70_1 = d69_1"
equation "d71_1 = d68_1"
equation "d73_1 = d72_1"
equation "d74_1 = 10 mm + 2 mm"
equation "d78_1 = d77_1 / 2"
equation "d79_1 = d78_1"
equation "d80_1 = d78_1"
equation "d81_1 = d78_1"
equation "d88_1 = d87_1"
equation "d89_1 = d87_1"
equation "d90_1 = d87_1"
equation "d108 = d103"
equation "d109 = d102"
equation "d122 = d121"
equation "d124 = d123"
equation "d128 = d127"
equation "d108_1 = d103_1"
equation "d109_1 = d102_1"
equation "d122_1 = d121_1"
equation "d124_1 = d123_1"
equation "d128_1 = d127_1"
equation "d140 = 160 mm + 10 mm"
equation "d142 = d140"
equation "d143 = d141"
equation "d146 = 10 mm - ( d141 / 2 )"
equation "d147 = d146"
